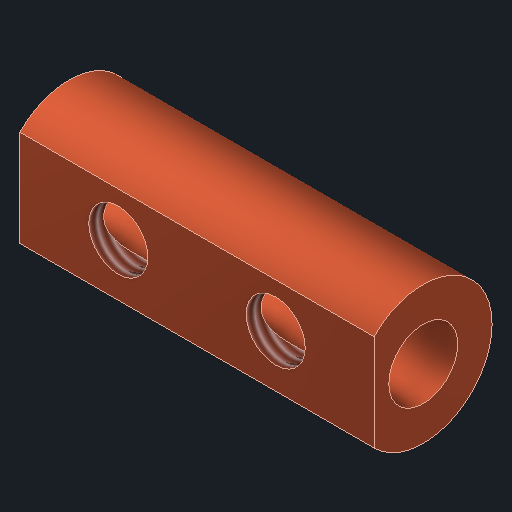
# Autodesk Inventor part: attachment2
Saved by Autodesk Inventor 2025 (Build 290162000, 162)
## iProperties
Created: 2023-12-08
Part Number: attachment2
Material: Generic
Document SubType Name: Modeling
Designer: jin20
Density: 1 g/cm^3
Appearance: 銅 - サテン
Author: jin20
Autodesk Inventor part; units mm, degrees
ref_plane "YZ Plane" through (0, 0, 0) normal (1, 0, 0) x (0, 1, 0)
ref_plane "XZ Plane" through (0, 0, 0) normal (0, 1, 0) x (-1, 0, 0)
ref_plane "XY Plane" through (0, 0, 0) normal (0, 0, 1) x (1, 0, 0)
sketch "スケッチ1" plane through (0, 0, 0) normal (1, 0, 0) x (0, 1, 0)
  circle A0 centre (0, 0) radius 3.5
  dimension "d0" = 7
  constraints: 1 centre point, 1 coincident
  measures "d0" diameter of A0
extrude "押し出し1" add sketch "スケッチ1" along normal mid plane 18
sketch "スケッチ2" plane through (9, 0, 0) normal (1, 0, 0) x (0, 0, -1)
  circle A0 centre (0, 0) radius 1.75
  dimension "d3" = 3.5
  constraints: 1 centre point, 1 coincident
  measures "d3" diameter of A0
extrude "押し出し2" cut sketch "スケッチ2" against normal through all
sketch "スケッチ3" plane through (9, 0, 0) normal (1, 0, 0) x (0, 0, -1)
  line L0 (-4.5, 4.5039) -> (-2.5, 4.5039)
  line L1 (-2.5, 4.5039) -> (-2.5, -4.5039)
  line L2 (-2.5, -4.5039) -> (-4.5, -4.5039)
  line L3 (-4.5, -4.5039) -> (-4.5, 4.5039)
  circle A0 centre (0, 0) radius 3.5 projected
  line L4 (-4.5, 4.5039) -> (-2.5, -4.5039) construction
  line L5 (-2.5, 4.5039) -> (-4.5, -4.5039) construction
  point P0 (-3.5, 0)
  constraints: 12 end point, 2 midpoint, 2 parallel, 1 horizontal, 1 horizontal alignment, 1 perpendicular, 1 other
extrude "押し出し3" cut sketch "スケッチ3" against normal through all contours L0 L1 A0 L2 L3 | L1 A0 picked at (-2.8262, -0.1289)
sketch "スケッチ5" plane through (9, -2.4495, 2.5) normal (0, 0, 1) x (1, 0, 0)
  circle A0 centre (-13, 2.6458) radius 1.5
  line L0 (-9, 2.4495) -> (-9, 9.8667) construction
  circle A1 centre (-5, 2.6458) radius 1.5
  dimension "d10" = 3
  constraints: 2 centre point, 2 end point, 1 symmetric about line, 1 vertical, 1 other
  measures "d10" diameter of A0
extrude "押し出し4" cut sketch "スケッチ5" against normal blind 3
thread "ねじ1" size "M3x0.5" class "6H" standard "ANSI Metric M Profile" full length
thread "ねじ2" size "M3x0.5" class "6H" standard "ANSI Metric M Profile" full length
